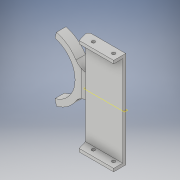
# Autodesk Inventor part: cameraMount
Saved by Autodesk Inventor 2018 (Build 220112000, 112)
## iProperties
Created: 2020-01-14
Part Number: cameraMount
Material: Generic
Document SubType Name: Modeling
Designer: anirudh.bali
Density: 1 g/cm^3
Appearance: Default
Author: anirudh.bali
Autodesk Inventor part; units mm, degrees
ref_plane "YZ Plane" through (0, 0, 0) normal (1, 0, 0) x (0, 1, 0)
ref_plane "XZ Plane" through (0, 0, 0) normal (0, 1, 0) x (-1, 0, 0)
ref_plane "XY Plane" through (0, 0, 0) normal (0, 0, 1) x (1, 0, 0)
sketch "Sketch1" plane through (0, 0, 0) normal (0, 1, 0) x (-1, 0, 0)
  circle A0 centre (0, 0) radius 1.75
  line L0 (-27.6489, -6.35) -> (8.2567, -6.35)
  line L1 (0, 6.35) -> (8.675, 6.35)
  circle A1 centre (-21.2989, 0) radius 1.75
  line L2 (-27.6489, 0) -> (-27.6489, 6.35)
  line L3 (-27.6489, 6.35) -> (0.5716, 6.35)
  line L4 (-27.6489, 0) -> (-27.6489, -6.35)
  arc A2 (8.2567, -6.35) -> (11.314, -2.3183) centre (8.2567, -3.175) ccw
  line L5 (-27.6489, -6.35) -> (8.2567, -6.35)
  arc A3 (8.2567, -6.35) -> (11.314, -2.3183) centre (8.2567, -3.175) ccw
  arc A4 (11.314, -2.3183) -> (8.675, 6.35) centre (-184.3483, -57.15) ccw
  constraints: 12 end point, 6 point on circle, 5 centre point, 3 point on line, 1 coincident, 1 perpendicular, 1 tangent
extrude "Extrusion1" add sketch "Sketch1" along normal blind 3.175
sketch "Sketch2" plane through (0, 3.175, 0) normal (0, 1, 0) x (1, 0, 0)
  line L0 (27.6489, 6.35) -> (-8.2567, 6.35) projected
  arc A0 (-8.2567, 6.35) -> (-11.314, 2.3183) centre (-8.2567, 3.175) ccw projected
  line L1 (27.6489, 6.35) -> (-8.2567, 6.35)
  line L2 (-11.4317, 3.175) -> (27.6489, 3.175)
  line L3 (27.6489, 3.175) -> (27.6489, 6.35)
  arc A1 (-8.2567, 6.35) -> (-11.4317, 3.175) centre (-8.2567, 3.175) ccw
  point P0 (0, 0)
  constraints: 7 end point, 3 point on circle, 1 centre point, 1 coincident, 1 horizontal, 1 parallel
extrude "Extrusion2" add sketch "Sketch2" along normal blind 47.625
ref_plane "Work Plane1" through (0, 50.8, 0) normal (0, 1, 0) x (1, 0, 0)
mirror "Mirror1" about plane through (0, 50.8, 0) normal (0, 1, 0) of "Extrusion1", "Extrusion2"
sketch "Sketch4" plane through (0, 50.8, 0) normal (0, 1, 0) x (1, 0, 0)
  line L0 (27.6489, 6.35) -> (-8.2567, 6.35) projected
  arc A0 (-19.3411, 37.8477) -> (27.6489, 6.35) centre (27.6489, 57.15) ccw
  line L1 (27.6489, 6.35) -> (-8.2567, 6.35)
  arc A1 (-19.3411, 16.3849) -> (-8.2567, 6.35) centre (27.6489, 57.15) ccw
  line L2 (-19.3411, 16.3849) -> (-19.3411, 37.8477)
  point P0 (0, 0)
  constraints: 5 point on circle, 4 end point, 2 centre point, 1 coincident, 1 vertical
extrude "Extrusion3" add sketch "Sketch4" along normal mid plane 25.4
ref_plane "Work Plane2" through (-19.3411, 50.8, -16.3849) normal (0, 0, 1) x (0, 1, 0)
sketch "Sketch6" plane through (-19.3411, 50.8, -16.3849) normal (0, 0, 1) x (0, 1, 0)
  line L0 (12.7, -11.0844) -> (12.7, 0) projected
  arc A0 (-27.6013, 27.5292) -> (27.6013, 27.5292) centre (0, 34.925) ccw
  line L1 (27.6013, 27.5292) -> (33.735, 25.8857)
  line L2 (0, 34.925) -> (53.4659, 34.925) construction
  line L3 (-27.6013, 27.5292) -> (-33.735, 25.8857)
  line L4 (0, 34.925) -> (52.592, 34.925) construction
  line L5 (12.7, 0) -> (12.7, 2.3909)
  line L6 (-12.7, 0) -> (12.7, 0) projected
  line L7 (12.7, 0) -> (-12.7, 0)
  line L8 (-12.7, 0) -> (-12.7, 2.3909)
  arc A1 (-33.735, 25.8857) -> (-12.7, 2.3909) centre (0, 34.925) ccw
  arc A2 (12.7, 2.3909) -> (33.735, 25.8857) centre (0, 34.925) ccw
  point P0 (-50.8, -19.3411)
  point P1 (0, 0)
  point P2 (0, 6.35)
  dimension "d17" = 6.35
  constraints: 14 end point, 7 point on circle, 3 centre point, 3 horizontal, 2 coincident, 1 perpendicular, 1 vertical
  measures "d17" distance of point (0, 0) point (0, 6.35)
sketch "Sketch7" plane through (0, 63.5, 0) normal (0, 1, 0) x (1, 0, 0)
  line L0 (-19.3411, 16.3849) -> (-19.3411, 37.8477) projected
  line L1 (-19.3411, 16.3849) -> (15.5035, 16.3849)
  line L2 (15.5035, 16.3849) -> (15.5035, 44.5768)
  line L3 (15.5035, 44.5768) -> (-19.3411, 44.5768)
  line L4 (-19.3411, 44.5768) -> (-19.3411, 16.3849)
  point P0 (0, 0)
  constraints: 8 end point, 2 parallel, 1 horizontal, 1 perpendicular
extrude "Extrusion5" cut sketch "Sketch7" against normal blind 43.942
sketch "Sketch8" plane through (0, 63.5, 0) normal (0, 1, 0) x (1, 0, 0)
  line L0 (-19.3411, 16.3849) -> (-19.3411, 6.3519) projected
  line L1 (-19.3411, 16.3849) -> (-19.3411, 6.35)
  arc A0 (-19.3411, 16.3849) -> (-8.2567, 6.35) centre (27.6489, 57.15) ccw projected
  line L2 (27.6489, 6.35) -> (-8.2567, 6.35) projected
  arc A1 (-19.3411, 16.3849) -> (-8.2567, 6.35) centre (27.6489, 57.15) ccw
  line L3 (27.6489, 6.35) -> (-8.2567, 6.35) projected
  line L4 (-19.3411, 6.35) -> (-8.2567, 6.35)
  line L5 (-19.3411, 6.35) -> (-19.3411, 16.3849)
  point P0 (0, 0)
  constraints: 8 end point, 2 point on circle, 2 point on line, 1 centre point, 1 collinear, 1 concentric, 1 horizontal, 1 vertical
extrude "Extrusion6" add sketch "Sketch8" against normal blind 25.4
extrude "Extrusion7" add sketch "Sketch6" along normal blind 10.033
fillet "Fillet1" radius 12.7 2 edges at (-21.7321, 63.5, -11.3684) (-21.7321, 38.1, -11.3684)
fillet "Fillet2" radius 6.35 1 edges at (-2.6636, 50.8, -16.3849)
body "Solid1"
